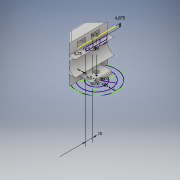
# Autodesk Inventor part: Stangenbereich_2
Saved by Autodesk Inventor 2018 (Build 220112000, 112)
## iProperties
Created: 2018-01-26
Part Number: Stangenbereich_2
Material: Generisch
Document SubType Name: Modeling
Designer: dreckWindof
Density: 1 g/cm^3
Appearance: Vorgabe
Author: dreckWindof
Autodesk Inventor part; units mm, degrees
sketch "Skizze1" plane through (0, 0, 0) normal (0, 0, 1) x (1, 0, 0)
  circle A0 centre (0, 0) radius 21
  line L0 (-16.8526, 12.5296) -> (0, 0)
  line L1 (0, 0) -> (-8.33, 19.2772)
  line L2 (0, 0) -> (8.0192, 19.4086)
  line L3 (0, 0) -> (18.1865, 10.5)
  line L4 (0, 0) -> (21, 0) construction
  line L5 (0, 0) -> (-13.5496, -16.044)
  line L6 (0, 0) -> (13.0769, -16.4315)
  circle A1 centre (0, 0) radius 27.5
  circle A2 centre (0, 0) radius 12.5
  line L7 (-27.5, 11.3909) -> (-11.3909, 27.5)
  line L8 (-11.3909, 27.5) -> (11.3909, 27.5)
  line L9 (11.3909, 27.5) -> (27.5, 11.3909)
  line L10 (27.5, 11.3909) -> (27.5, -11.3909)
  line L11 (27.5, -11.3909) -> (11.3909, -27.5)
  line L12 (11.3909, -27.5) -> (-11.3909, -27.5)
  line L13 (-11.3909, -27.5) -> (-27.5, -11.3909)
  line L14 (-27.5, -11.3909) -> (-27.5, 11.3909)
  circle A3 centre (0, 0) radius 3.25
  point P0 (0, 0)
  point P1 (-27.5, 0)
  dimension "d3" = 55
  dimension "d0" = 42
  dimension "d1" = 30
  dimension "d2" = 30
  dimension "d4" = 25
  dimension "d27" = 0
  dimension "d28" = 0
  dimension "d105" = 6.5
  constraints: 30 end point, 6 point on circle, 4 coincident, 3 centre point, 1 equal length, 1 horizontal, 1 horizontal alignment, 1 midpoint, 19 other
  measures "d0" diameter of A0
  measures "d1" angle of L1 L0
  measures "d2" angle of L4 L3
  measures "d4" diameter of A2
  measures "d27" distance of point (0, 0) L0.end
  measures "d28" distance of L0.end point (0, 0)
  measures "d105" diameter of A3
extrude "Extrusion21" add sketch "Skizze1" along normal blind 53 contours A0 L6 A2 L3 | L3 A2 L2 A0 | A0 L5 A2 L6 | L2 A2 L1 A0 | A2 L6 A3 L3 | L3 A3 L2 A2 | A0 L0 A2 L5 | A2 L5 A3 L6 | L1 A2 L0 A0 | L2 A3 L1 A2 | A3 L6 L3 | L3 L2 A3 | A2 L0 A3 L5 | A3 L5 L6 | L1 A3 L0 A2 | L2 L1 A3 | L5 A3 L0 | L0 A3 L1 | A1 | L10 L11 A1 | A1 L9 L10 | A1 L8 L9 | L11 L12 A1 | A1 L7 L8 | L12 L13 A1 | A1 L14 L7 | L13 L14 A1
sketch "Skizze18" plane through (0, 0, 0) normal (0, 0, 1) x (1, 0, 0)
  line L0 (-11.3909, 27.5) -> (11.3909, 27.5) projected
  line L1 (-11.3909, 27.5) -> (63.1653, 27.5)
  line L2 (63.1653, 27.5) -> (63.1653, -27.5)
  line L3 (63.1653, -27.5) -> (-11.3909, -27.5)
  line L4 (-11.3909, -27.5) -> (-11.3909, 27.5)
  point P0 (0, 0)
  dimension "d154" = 55
  constraints: 8 end point, 2 parallel, 1 horizontal, 1 perpendicular
  measures "d154" distance of L1.end L2.end
extrude "Extrusion22" cut sketch "Skizze18" along normal through all
sketch "Skizze19" plane through (0, 0, 0) normal (1, 0, 0) x (0, 1, 0)
  line L0 (12.25, 9.875) -> (-12.25, 9.875)
  line L1 (-12.25, 9.875) -> (-12.25, 5.125)
  line L2 (-12.25, 5.125) -> (12.25, 5.125)
  line L3 (12.25, 5.125) -> (12.25, 9.875)
  line L4 (27.5, 0) -> (-27.5, 0) projected
  line L5 (-27.5, 0) -> (-27.5, 53) projected
  point P0 (0, 0)
  dimension "d157" = 24.5
  dimension "d158" = 4.75
  dimension "d159" = 5.125
  dimension "d160" = 39.75
  constraints: 8 end point, 2 parallel, 1 horizontal, 1 perpendicular
  measures "d157" distance of L2.end L1.end
  measures "d158" distance of L1.end L0.end
  measures "d159" distance from line of L4 L2.end
  measures "d160" distance from line of L5 L0.start
sketch "Skizze20" plane through (0, 0, 0) normal (1, 0, 0) x (0, 1, 0)
  line L0 (-15, 48.125) -> (15, 48.125)
  line L1 (15, 48.125) -> (15, 42.875)
  line L2 (15, 42.875) -> (-15, 42.875)
  line L3 (-15, 42.875) -> (-15, 48.125)
  line L4 (5, 48.125) -> (-5, 48.125)
  line L5 (-5, 48.125) -> (-5, 42.875)
  line L6 (-5, 42.875) -> (5, 42.875)
  line L7 (5, 42.875) -> (5, 48.125)
  line L8 (-27.5, 53) -> (27.5, 53) projected
  point P0 (0, 0)
  dimension "d165" = 30
  dimension "d166" = 5.25
  dimension "d168" = 10
  dimension "d169" = 5.25
  dimension "d170" = 10
  dimension "d171" = 5
  dimension "d172" = 4.875
  constraints: 16 end point, 4 parallel, 2 horizontal, 2 perpendicular, 1 point on line
  measures "d165" distance of L1.end L2.end
  measures "d166" distance of L2.end L0.start
  measures "d168" distance of L6.end L5.end
  measures "d169" distance of L4.end L5.end
  measures "d170" distance of L2.end L5.end
  measures "d171" horizontal distance of point (0, 0) L5.end
  measures "d172" distance from line of L8 L0.end
extrude "Extrusion23" cut sketch "Skizze20" against normal blind 20.5 contours L0 L5 L2 L3 | L0 L1 L2 L7
extrude "Extrusion25" add sketch "Skizze19" along normal blind 10 and the other way blind 25
fillet "Rundung11" radius 2 5 edges at (-19.4454, 19.4454, 53) (-27.5, 0, 53) (-19.4454, -19.4454, 53) (-27.5, -11.3909, 26.5) (-27.5, 11.3909, 26.5)
fillet "Rundung12" radius 1 12 edges at (-11.3909, 15, 45.5) (-11.3909, 10, 42.875) (-11.3909, 5, 45.5) (-11.3909, 10, 48.125) (-11.3909, -5, 45.5) (-11.3909, -10, 42.875) (-11.3909, -15, 45.5) (-11.3909, -10, 48.125) (10, 0, 9.875) (10, -12.25, 7.5) (10, 0, 5.125) (10, 12.25, 7.5)
sketch "Skizze22" plane through (0, 0, 0) normal (0, 1, 0) x (-1, 0, 0)
  line L0 (26.9142, 0) -> (11.3909, 0) projected
  line L1 (11.3909, 0) -> (11.3909, 51) projected
  line L2 (11.3909, 53) -> (25.5, 53) projected
  line L3 (-11.1091, 37.75) -> (-11.1091, 15.25)
  line L4 (11.3909, 15.25) -> (11.3909, 37.75)
  line L5 (11.3909, 37.75) -> (2.2757, 37.75)
  line L6 (-2.494, 37.75) -> (-11.1091, 37.75)
  arc A0 (-2.494, 37.75) -> (-2.494, 15.25) centre (-0.1091, 26.5) ccw
  arc A1 (2.2757, 15.25) -> (2.2757, 37.75) centre (-0.1091, 26.5) ccw
  line L7 (-11.1091, 15.25) -> (-2.494, 15.25)
  line L8 (2.2757, 15.25) -> (11.3909, 15.25)
  line L9 (11.3909, 0) -> (11.3909, 51) projected
  point P0 (0, 0)
  point P1 (11.3909, 26.5)
  dimension "d195" = 26.5
  dimension "d196" = 11.5
  dimension "d197" = 22.5
  dimension "d198" = 22.5
  dimension "d199" = 15.25
  dimension "d200" = 0
  constraints: 12 end point, 5 parallel, 5 point on circle, 3 coincident, 2 centre point, 2 horizontal, 2 perpendicular, 1 point on line
  measures "d195" distance from line of L2 A0.centre
  measures "d196" distance from line of L1 A0.centre
  measures "d197" distance of L4.start L3.end
  measures "d198" distance of L3.end L3.start
  measures "d199" distance from line of L2 L4.end
  measures "d200" distance from line of L1 L4.end
extrude "Extrusion26" cut sketch "Skizze1" along normal blind 20 contours A3 L6 L3 | L3 L2 A3 | A3 L5 L6 | L2 L1 A3 | L5 A3 L0 | L0 A3 L1
extrude "Extrusion28" add sketch "Skizze22" along normal mid plane 55 contours L8 A1 L1 | A1 L5 L1
sketch "Skizze12" plane through (0, 0, 14.5) normal (0, 0, 1) x (1, 0, 0)
  circle A0 centre (0, 0) radius 21
  line L0 (-16.8526, 12.5296) -> (-10.0313, 7.4581)
  line L1 (-4.9583, 11.4745) -> (-8.33, 19.2772)
  line L2 (4.7734, 11.5527) -> (8.0192, 19.4086)
  line L3 (10.8253, 6.25) -> (18.1865, 10.5)
  line L4 (0, 0) -> (21, 0) construction
  line L5 (-8.0652, -9.55) -> (-13.5496, -16.044)
  line L6 (7.7839, -9.7807) -> (13.0769, -16.4315)
  circle A1 centre (0, 0) radius 27.5
  circle A2 centre (0, 0) radius 12.5
  line L7 (-27.5, 11.3909) -> (-11.3909, 27.5)
  line L8 (-11.3909, 27.5) -> (11.3909, 27.5)
  line L9 (11.3909, 27.5) -> (27.5, 11.3909)
  line L10 (27.5, 11.3909) -> (27.5, -11.3909)
  line L11 (27.5, -11.3909) -> (11.3909, -27.5)
  line L12 (11.3909, -27.5) -> (-11.3909, -27.5)
  line L13 (-11.3909, -27.5) -> (-27.5, -11.3909)
  line L14 (-27.5, -11.3909) -> (-27.5, 11.3909)
  point P0 (0, 0)
  point P1 (-27.5, 0)
  dimension "d91" = 55
  dimension "d88" = 42
  dimension "d89" = 30
  dimension "d90" = 30
  dimension "d92" = 25
  dimension "d93" = 0
  dimension "d94" = 0
  constraints: 30 end point, 12 point on circle, 3 coincident, 2 centre point, 1 horizontal, 1 horizontal alignment, 1 midpoint, 19 other
  measures "d88" diameter of A0
  measures "d89" angle of L1 L0
  measures "d90" angle of L4 L3
  measures "d92" diameter of A2
  measures "d93" distance of point (0, 0) L4.start
  measures "d94" distance of L4.start point (0, 0)
sketch "Skizze13" plane through (0, -27.5, 0) normal (0, 1, 0) x (-1, 0, 0)
  circle A0 centre (0, 41) radius 11.5
  line L0 (-38.5, 14.5) -> (38.5, 14.5) projected
  line L1 (27.5, 0) -> (27.5, 67.5) projected
  point P0 (0, 0)
  point P1 (27.5, 14.5)
  dimension "d100" = 23
  dimension "d101" = 26.5
  dimension "d102" = 27.5
  constraints: 1 centre point
  measures "d100" diameter of A0
  measures "d101" distance from line of L0 A0.centre
  measures "d102" distance from line of L1 A0.centre
sketch "Skizze14" plane through (0, 0, 0) normal (0, 1, 0) x (-1, 0, 0)
  line L0 (11.3909, 42.5805) -> (11.3909, 39.4195) projected
  line L1 (27.5, 67.5) -> (11.3909, 67.5)
  line L2 (11.3909, 67.5) -> (11.3909, 14.5)
  line L3 (11.3909, 14.5) -> (27.5, 14.5)
  line L4 (27.5, 14.5) -> (27.5, 67.5)
  arc A0 (11.3909, 42.5805) -> (-11.3909, 42.5805) centre (0, 41) ccw projected
  line L5 (0, 52.5) -> (11.3909, 52.5)
  line L6 (11.3909, 52.5) -> (11.3909, 29.5)
  line L7 (11.3909, 29.5) -> (0, 29.5)
  line L8 (0, 29.5) -> (0, 52.5)
  point P0 (0, 0)
  dimension "d108" = 23
  dimension "d111" = 25
  dimension "d112" = 5.25
  dimension "d113" = 5.375
  dimension "d114" = 40
  dimension "d115" = 30
  dimension "d116" = 4.75
  dimension "d117" = 4.875
  dimension "d124" = 10
  dimension "d125" = 4.75
  dimension "d126" = 10
  constraints: 24 end point, 6 parallel, 3 horizontal, 3 perpendicular, 1 point on line
  measures "d111" distance of L1.end L2.end
  measures "d112" distance of L2.end L0.start
  measures "d113" distance from line of L4 L2.end
  measures "d114" distance from line of L5 L2.end
  measures "d115" distance of L7.end L8.end
  measures "d116" distance of L8.end L6.start
sketch "Skizze16" plane through (-11.391, 0, 0) normal (1, 0, 0) x (0, 1, 0)
  line L0 (-12.5, 25.125) -> (12.5, 25.125)
  line L1 (12.5, 25.125) -> (12.5, 19.875)
  line L2 (12.5, 19.875) -> (-12.5, 19.875)
  line L3 (-12.5, 19.875) -> (-12.5, 25.125)
  line L4 (-15, 62.125) -> (15, 62.125)
  line L5 (15, 62.125) -> (15, 57.375)
  line L6 (15, 57.375) -> (-15, 57.375)
  line L7 (-15, 57.375) -> (-15, 62.125)
  line L8 (5, 62.125) -> (-5, 62.125)
  line L9 (-5, 62.125) -> (-5, 57.375)
  line L10 (-5, 57.375) -> (5, 57.375)
  line L11 (5, 57.375) -> (5, 62.125)
  point P0 (0, 0)
  dimension "d130" = 25
  dimension "d131" = 5.25
  dimension "d134" = 30
  dimension "d135" = 4.75
  dimension "d137" = 10
  dimension "d138" = 4.75
  dimension "d139" = 10
  dimension "d144" = 42
  dimension "d145" = 30
  dimension "d146" = 30
  dimension "d148" = 25
  dimension "d149" = 0
  dimension "d150" = 0
  dimension "d151" = 6.5
  constraints: 30 end point, 6 point on circle, 4 coincident, 3 centre point, 1 equal length, 1 horizontal, 1 horizontal alignment, 1 midpoint, 19 other
  measures "d145" angle of L1 L0
  measures "d146" angle of L4 L3
  measures "d149" distance of point (0, 0) L0.end
  measures "d150" distance of L0.end point (0, 0)
sketch "Skizze2" plane through (0, 0, 14.5) normal (0, 0, 1) x (1, 0, 0)
  circle A0 centre (0, 0) radius 21
  line L0 (-16.8526, 12.5296) -> (0, 0)
  line L1 (0, 0) -> (-8.33, 19.2772)
  line L2 (0, 0) -> (8.0192, 19.4086)
  line L3 (0, 0) -> (18.1865, 10.5)
  line L4 (0, 0) -> (21, 0) construction
  line L5 (0, 0) -> (-13.5496, -16.044)
  line L6 (0, 0) -> (13.0769, -16.4315)
  circle A1 centre (0, 0) radius 27.5
  circle A2 centre (0, 0) radius 12.5
  point P0 (0, 0)
  dimension "d11" = 42
  dimension "d12" = 30
  dimension "d13" = 30
  dimension "d14" = 55
  dimension "d15" = 25
  dimension "d29" = 0
  dimension "d30" = 0
  constraints: 14 end point, 6 point on circle, 3 centre point, 2 coincident, 1 equal length, 1 horizontal
  measures "d11" diameter of A0
  measures "d12" angle of L1 L0
  measures "d13" angle of L4 L3
  measures "d14" diameter of A1
  measures "d15" diameter of A2
  measures "d29" distance of point (0, 0) L0.end
  measures "d30" distance of point (0, 0) L0.end
sketch "Skizze3" plane through (0, 0, 48) normal (0, 0, 1) x (1, 0, 0)
  circle A0 centre (0, 0) radius 3.25
  dimension "d19" = 6.5
  dimension "d38" = 0
  constraints: 1 centre point
  measures "d19" diameter of A0
  measures "d38" distance of point (0, 0) A0.centre
sketch "Skizze6" plane through (0, 0, 14.5) normal (0, 0, 1) x (1, 0, 0)
  circle A0 centre (0, 0) radius 21
  line L0 (-16.8526, 12.5296) -> (0, 0)
  line L1 (0, 0) -> (-8.33, 19.2772)
  line L2 (0, 0) -> (8.0192, 19.4086)
  line L3 (0, 0) -> (18.1865, 10.5)
  line L4 (0, 0) -> (21, 0) construction
  line L5 (0, 0) -> (-13.5496, -16.044)
  line L6 (0, 0) -> (13.0769, -16.4315)
  circle A1 centre (0, 0) radius 27.5
  circle A2 centre (0, 0) radius 12.5
  line L7 (5.2672, -3.0014) -> (0.0343, -6.0622)
  line L8 (0.0343, -6.0622) -> (-5.2328, -3.0608)
  line L9 (-5.2328, -3.0608) -> (-5.2672, 3.0014)
  line L10 (-5.2672, 3.0014) -> (-0.0343, 6.0622)
  line L11 (-0.0343, 6.0622) -> (5.2328, 3.0608)
  line L12 (5.2328, 3.0608) -> (5.2672, -3.0014)
  point P0 (0, 0)
  dimension "d31" = 42
  dimension "d32" = 30
  dimension "d33" = 30
  dimension "d34" = 55
  dimension "d35" = 25
  dimension "d36" = 0
  dimension "d37" = 0
  dimension "d39" = 10.5
  constraints: 26 end point, 6 point on circle, 3 centre point, 3 coincident, 1 equal length, 1 horizontal, 13 other
  measures "d31" diameter of A0
  measures "d32" angle of L1 L0
  measures "d33" angle of L4 L3
  measures "d34" diameter of A1
  measures "d35" diameter of A2
  measures "d36" distance of point (0, 0) L0.end
  measures "d37" distance of L0.end point (0, 0)
  measures "d39" horizontal distance of L8.end L7.start
sketch "Skizze7" plane through (0, 0, 48) normal (0, 0, 1) x (1, 0, 0)
  circle A0 centre (0, 0) radius 27.5 projected
  line L0 (27.5, -11.3909) -> (11.3909, -27.5)
  line L1 (11.3909, -27.5) -> (-11.3909, -27.5)
  line L2 (-11.3909, -27.5) -> (-27.5, -11.3909)
  line L3 (-27.5, -11.3909) -> (-27.5, 11.3909)
  line L4 (-27.5, 11.3909) -> (-11.3909, 27.5)
  line L5 (-11.3909, 27.5) -> (11.3909, 27.5)
  line L6 (11.3909, 27.5) -> (27.5, 11.3909)
  line L7 (27.5, 11.3909) -> (27.5, -11.3909)
  point P0 (0, 0)
  point P1 (0, 0)
  point P2 (27.5, 0)
  dimension "d45" = 23
  dimension "d46" = 16.5
  dimension "d47" = 43.125
  constraints: 1 centre point
  measures "d45" diameter of A0
  measures "d46" distance from line of L0 A0.centre
  measures "d47" distance from line of L1 A0.centre
sketch "Skizze9" plane through (27.5, -11.3909, 48) normal (1, 0, 0) x (0, 0, -1)
  circle A0 centre (16.5, 27.0159) radius 9.5
  line L0 (0, 22.7817) -> (0, 0) projected
  line L1 (0, -16.1091) -> (48, -16.1091) projected
  point P0 (-48, 11.3909)
  dimension "d49" = 19
  dimension "d52" = 16.5
  dimension "d53" = 43.125
  constraints: 1 centre point
  measures "d49" diameter of A0
  measures "d52" distance from line of L0 A0.centre
  measures "d53" distance from line of L1 A0.centre
sketch "Skizze10" plane through (27.5, -11.3909, 48) normal (1, 0, 0) x (0, 0, -1)
  line L0 (25, 43.6027) -> (8, 43.6027)
  line L1 (8, 43.6027) -> (8, 26.6027)
  line L2 (8, 26.6027) -> (25, 26.6027)
  line L3 (25, 26.6027) -> (25, 43.6027)
  ellipse E0 centre (16.5, 26.6027) end of major axis (16.5, 37.9638) minor radius 11.3535 (27.1922, 22.7817) -> (5.8078, 22.7817) ccw projected
  point P0 (48, 11.3909)
  dimension "d58" = 17
  dimension "d59" = 17
  dimension "d60" = 17
  dimension "d61" = 8.5
  constraints: 8 end point, 2 parallel, 1 horizontal, 1 perpendicular, 1 other
  measures "d58" distance of L2.end L1.end
  measures "d59" distance of L1.end L0.end
  measures "d60" vertical distance of point (16.5, 26.603) L0.start
  measures "d61" horizontal distance of point (16.5, 26.603) L0.end
equation "\"d169\" = d166"
equation "\"d171\" = 0.5 * d168"
equation "\"d196\" = 0.5 * d194"
equation "\"d125\" = d116"
equation "\"d138\" = d135"
equation "\"d52\" = d46"
equation "\"d53\" = d47"
equation "\"d194\" = 23"
